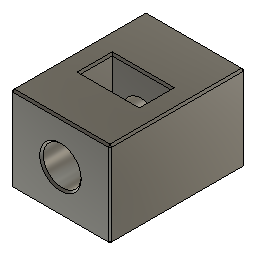
Hilfsanschlag Einsatzmutter klein v2 (Autodesk Fusion 360 design; units mm, degrees)
Autodesk Fusion 360 part; units mm, degrees
sketch "Sketch1" plane through (0, 0, 0) normal (0, 1, 0) x (1, 0, 0)
  line L0 (0, 0) -> (22, 0)
  line L1 (22, 0) -> (22, -19)
  line L2 (22, -19) -> (0, -19)
  line L3 (0, -19) -> (0, 0)
  line L4 (0, -9.5) -> (22, -9.5) construction
  line L5 (17.5, -13.2528) -> (17.5, -5.7472)
  line L6 (17.5, -5.7472) -> (11, -1.9944)
  line L7 (11, -1.9944) -> (4.5, -5.7472)
  line L8 (4.5, -5.7472) -> (4.5, -13.2528)
  line L9 (4.5, -13.2528) -> (11, -17.0056)
  line L10 (11, -17.0056) -> (17.5, -13.2528)
  line L11 (17.5, -13.2528) -> (17.5, -19)
  line L12 (4.5, -13.2528) -> (4.5, -19)
  circle A0 centre (11, -9.5) radius 4.2
  point P0 (11, -9.5)
  dimension "d1" = 19
  dimension "d2" = 22
  dimension "d3" = 13
  dimension "d4" = 8.4
  constraint horizontal L0
  constraint vertical L1
  constraint horizontal L2
  constraint vertical L3
  constraint coincident L0.start L3.end
  constraint midpoint L3 L4.start
  constraint midpoint L1 L4.end
  constraint midpoint L4 P0
  constraint vertical L5
  constraint parallel L5 L11
  constraint coincident L2 L12.end
  constraint perpendicular L2 L12
  constraint coincident P0 A0.centre
  measures "d1" distance of L0.end L1.end
  measures "d2" distance of L1.end L2.end
  measures "d3" distance of L5 L8
  measures "d4" diameter of A0
extrude "Extrude1" add sketch "Sketch1" along normal blind 30
extrude "Extrude2" cut sketch "Sketch1" along normal blind 7 from surface at 11 contours L2 L9 L10 L11 L12 | L5 L6 L7 L8 L9 L10
chamfer "Chamfer1" distance 0.4 angle 45 18 edges at (0, 15, 19) (0, 15, 0) (22, 15, 19) (22, 15, 0) (22, 30, 9.5) (11, 30, 19) (0, 30, 9.5) (11, 30, 0) (22, 0, 9.5) (11, 0, 19) (11, 0, 0) (0, 0, 9.5) (4.5, 14.5, 19) (17.5, 14.5, 19) (7.0842, 0, 7.9812) (7.0842, 30, 7.9812) (11, 18, 19) (11, 11, 19)
